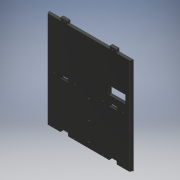
# Autodesk Inventor part: BA04
Saved by Autodesk Inventor 2017 (Build 210142000, 142)
## iProperties
Created: 2019-05-22
Part Number: BA04
Material: Wood (Cherry)
Document SubType Name: Modeling
Designer: Dell
Density: 0.63 g/cm^3
Appearance: Smooth - Black
Mass: 791.209 g
Surface Area: 2249.26 cm^2
Volume: 1255.89 cm^3
Author: Dell
Autodesk Inventor part; units mm, degrees
ref_plane "YZ Plane" through (0, 0, 0) normal (1, 0, 0) x (0, 1, 0)
ref_plane "XZ Plane" through (0, 0, 0) normal (0, 1, 0) x (-1, 0, 0)
ref_plane "XY Plane" through (0, 0, 0) normal (0, 0, 1) x (1, 0, 0)
sketch "Sketch1" plane through (0, 0, 0) normal (0, 0, 1) x (1, 0, 0)
  line L0 (0, 0) -> (303.5592, 0)
  line L1 (303.5592, 0) -> (455.3388, -262.89) construction
  line L2 (455.3388, -262.89) -> (404.5388, -350.8782)
  line L3 (404.5388, -350.8782) -> (-50.8, -87.9882) construction
  line L4 (-50.8, -87.9882) -> (0, 0) construction
  line L5 (0, 0) -> (5.4993, -9.525)
  line L6 (5.4993, -9.525) -> (298.06, -9.525)
  line L7 (298.06, -9.525) -> (303.5592, 0)
  dimension "d0" = 525.78
  dimension "d1" = 101.6
  dimension "d2" = 120
  dimension "d3" = 9.525
  dimension "d4" = 60
  dimension "d5" = 60
  constraints: 16 end point, 2 equal length, 2 horizontal, 2 perpendicular
  measures "d0" distance of L2.end L3.end
  measures "d1" distance of L3.end L0.start
  measures "d2" angle of L0 L4
  measures "d3" distance between parallel lines of L0 L6
  measures "d4" angle of L0 L5
  measures "d5" angle of L0 L7
extrude "Extrusion1" add sketch "Sketch1" along normal blind 346.075
sketch "Sketch2" plane through (5.4993, -9.525, 0) normal (0, -1, 0) x (1, 0, 0)
  line L0 (298.06, 346.075) -> (-5.4993, 346.075) projected
  line L1 (45.3007, 346.075) -> (70.7007, 346.075)
  line L2 (70.7007, 346.075) -> (70.7007, 355.6)
  line L3 (70.7007, 355.6) -> (45.3007, 355.6)
  line L4 (45.3007, 355.6) -> (45.3007, 346.075)
  line L5 (221.86, 346.075) -> (247.26, 346.075)
  line L6 (247.26, 346.075) -> (247.26, 355.6)
  line L7 (247.26, 355.6) -> (221.86, 355.6)
  line L8 (221.86, 355.6) -> (221.86, 346.075)
  line L9 (-5.4993, 0) -> (-5.4993, 346.075) projected
  line L10 (298.06, 0) -> (298.06, 346.075) projected
  circle A0 centre (58.0007, 350.8375) radius 2.25
  circle A1 centre (234.56, 350.8375) radius 2.25
  point P0 (58.0007, 355.6)
  point P1 (234.56, 355.6)
  point P2 (70.7007, 350.8375)
  point P3 (247.26, 350.8375)
  dimension "d8" = 25.4
  dimension "d9" = 9.525
  dimension "d10" = 25.4
  dimension "d11" = 9.525
  dimension "d12" = 50.8
  dimension "d13" = 50.8
  dimension "d16" = 4.5
  dimension "d17" = 4.5
  constraints: 16 end point, 4 midpoint, 4 parallel, 2 centre point, 2 horizontal, 2 horizontal alignment, 2 perpendicular, 2 point on line, 2 vertical alignment
  measures "d8" distance of L3.end L2.end
  measures "d9" distance of L2.end L1.end
  measures "d10" distance of L7.end L6.end
  measures "d11" distance of L6.end L5.end
  measures "d12" distance between parallel lines of L9 L4
  measures "d13" distance between parallel lines of L10 L6
  measures "d16" diameter of A0
  measures "d17" diameter of A1
extrude "Extrusion2" add sketch "Sketch2" against normal blind 9.525
ref_plane "Work Plane1" through (0, 0, 295.275) normal (0, 0, 1) x (1, 0, 0)
sketch "Sketch3" plane through (0, 0, 295.275) normal (0, 0, 1) x (1, 0, 0)
  line L0 (0, 0) -> (303.5592, 0) projected
  line L1 (0, 0) -> (0, -9.525)
  line L2 (298.06, -9.525) -> (5.4993, -9.525) projected
  line L3 (0, -9.525) -> (5.4993, -9.525)
  line L4 (5.4993, -9.525) -> (0, 0) projected
  constraints: 4 end point, 1 perpendicular, 1 vertical
extrude "Extrusion3" [suppressed]
ref_plane "Work Plane2" through (0, 0, 50.8) normal (0, 0, -1) x (-1, 0, 0)
sketch "Sketch4" plane through (0, 0, 50.8) normal (0, 0, -1) x (-1, 0, 0)
  line L0 (0, -12.7) -> (0, 0) projected
  line L1 (-7.3323, -12.7) -> (0, 0) projected
  line L2 (-7.3323, -12.7) -> (0, -12.7) projected
extrude "Extrusion4" [suppressed]
ref_plane "Work Plane3" through (0, 0, 173.0375) normal (0, 0, -1) x (-1, 0, 0)
sketch "Sketch5" plane through (0, 0, 173.0375) normal (0, 0, -1) x (-1, 0, 0)
  line L0 (0, 0) -> (0, -12.7) projected
  line L1 (0, -12.7) -> (-7.3323, -12.7) projected
  line L2 (0, 0) -> (-7.3323, -12.7) projected
extrude "Extrusion5" [suppressed]
ref_plane "Work Plane4" through (151.7796, -9.525, 346.075) normal (-1, 0, 0) x (0, 0, 1)
mirror "Mirror1" [suppressed]
sketch "Sketch6" plane through (0, 0, 0) normal (0, 0, -1) x (-1, 0, 0)
  line L0 (-76.9796, -9.525) -> (-76.9796, 0)
  line L1 (-76.9796, -4.7625) -> (-64.2796, -4.7625) construction
  circle A0 centre (-64.2796, -4.7625) radius 2.25
  line L2 (-64.2796, -4.7625) -> (-64.2796, 0) construction
  line L3 (-51.5796, -9.525) -> (-76.9796, -9.525)
  line L4 (-76.9796, 0) -> (-51.5796, 0)
  line L5 (-51.5796, 0) -> (-51.5796, -9.525)
  line L6 (-226.5796, 0) -> (-226.5796, -9.525)
  line L7 (-239.2796, 0) -> (-64.2796, 0) construction
  line L8 (-251.9796, 0) -> (-226.5796, 0)
  line L9 (-251.9796, -9.525) -> (-251.9796, 0)
  circle A1 centre (-239.2796, -4.7625) radius 2.25
  line L10 (-239.2796, -4.7625) -> (-239.2796, 0) construction
  line L11 (-239.2796, -4.7625) -> (-226.5796, -4.7625) construction
  line L12 (-226.5796, -9.525) -> (-251.9796, -9.525)
  line L13 (0, 0) -> (-303.5592, 0)
  line L14 (0, 0) -> (-303.5592, 0) projected
  line L15 (-298.06, -9.525) -> (-5.4993, -9.525) projected
  point P0 (-151.7796, 0)
  dimension "d26" = 25.4
  dimension "d29" = 25.4
  dimension "d30" = 175
  dimension "d31" = 4.5
  dimension "d32" = 4.5
  constraints: 28 end point, 7 midpoint, 6 perpendicular, 6 point on line, 4 parallel, 2 centre point
  measures "d26" distance of L0.end L5.start
  measures "d29" distance of L8.start L6.start
  measures "d30" distance of L7.start L2.end
  measures "d31" diameter of A1
  measures "d32" diameter of A0
extrude "Extrusion6" cut sketch "Sketch6" against normal blind 9.525 contours L0 L4 L5 L3 | L12 L9 L8 L6 | A0 | A1
sketch "Sketch7" plane through (227.3592, -9.525, 355.6) normal (0, -1, 0) x (1, 0, 0)
  line L0 (-175.7796, -178.275) -> (-150.3796, -178.275)
  line L1 (-150.3796, -178.275) -> (-150.3796, -187.8)
  line L2 (-150.3796, -187.8) -> (-175.7796, -187.8)
  line L3 (-175.7796, -187.8) -> (-175.7796, -178.275)
  line L4 (-0.7796, -178.275) -> (24.6204, -178.275)
  line L5 (24.6204, -178.275) -> (24.6204, -187.8)
  line L6 (24.6204, -187.8) -> (-0.7796, -187.8)
  line L7 (-0.7796, -187.8) -> (-0.7796, -178.275)
  line L8 (-175.7796, -346.075) -> (-150.3796, -346.075) projected
  line L9 (-0.7796, -346.075) -> (24.6204, -346.075) projected
  line L10 (-221.86, -9.525) -> (-176.5592, -9.525) projected
  point P0 (-227.3592, -355.6)
  point P1 (-163.0796, -187.8)
  point P2 (-163.0796, -346.075)
  point P3 (11.9204, -187.8)
  point P4 (11.9204, -346.075)
  dimension "d36" = 25.4
  dimension "d37" = 9.525
  dimension "d38" = 25.4
  dimension "d39" = 9.525
  dimension "d100" = 168.75
  constraints: 16 end point, 4 midpoint, 4 parallel, 2 horizontal, 2 perpendicular, 2 vertical alignment, 1 horizontal alignment
  measures "d36" distance of L1.end L2.end
  measures "d37" distance of L0.end L1.end
  measures "d38" distance of L5.end L6.end
  measures "d39" distance of L4.end L5.end
  measures "d100" distance between parallel lines of L10 L0
extrude "Extrusion7" cut sketch "Sketch7" against normal through all
sketch "Sketch8" plane through (227.3592, -9.525, 355.6) normal (0, -1, 0) x (1, 0, 0)
  line L0 (-150.3796, -355.6) -> (-0.7796, -355.6) construction
  line L1 (-100.9796, -355.6) -> (-50.1796, -355.6) construction
  line L2 (-50.1796, -355.6) -> (-50.1796, -178.275) construction
  line L3 (-50.1796, -178.275) -> (-100.9796, -178.275) construction
  line L4 (-100.9796, -178.275) -> (-100.9796, -355.6) construction
  circle A0 centre (-75.5796, -267.89) radius 4
  circle A1 centre (-75.5796, -200.18) radius 4
  circle A2 centre (-75.5796, -335.6) radius 4
  line L5 (-0.7796, -355.6) -> (-150.3796, -355.6)
  line L6 (-0.7796, -355.6) -> (-150.3796, -355.6) projected
  circle A3 centre (-126.3796, -183.0375) radius 2.25
  circle A4 centre (-126.3796, -350.8375) radius 2.25
  circle A5 centre (-24.7796, -350.8375) radius 2.25
  circle A6 centre (-24.7796, -183.0375) radius 2.25
  line L7 (-150.3796, -178.275) -> (-150.3796, -187.8) projected
  line L8 (-150.3796, -346.075) -> (-150.3796, -355.6) projected
  point P0 (-75.5796, -355.6)
  point P1 (-75.5796, -355.6)
  point P2 (-75.5796, -355.6)
  point P3 (-100.9796, -266.9375)
  point P4 (-150.3796, -183.0375)
  point P5 (-150.3796, -350.8375)
  dimension "d44" = 8
  dimension "d45" = 8
  dimension "d46" = 8
  dimension "d48" = 20
  dimension "d49" = 50.8
  dimension "d59" = 4.5
  dimension "d60" = 4.5
  dimension "d61" = 4.5
  dimension "d62" = 4.5
  dimension "d63" = 25.4
  dimension "d64" = 25.4
  dimension "d98" = 67.71
  dimension "d99" = 67.71
  constraints: 12 end point, 7 centre point, 7 midpoint, 5 horizontal alignment, 5 vertical alignment, 2 coincident, 2 parallel, 1 horizontal, 1 perpendicular, 1 point on line
  measures "d44" diameter of A0
  measures "d45" diameter of A1
  measures "d46" diameter of A2
  measures "d48" distance from line of L0 A2.centre
  measures "d49" distance of L2.end L3.end
  measures "d59" diameter of A3
  measures "d60" diameter of A4
  measures "d61" diameter of A5
  measures "d62" diameter of A6
  measures "d63" distance from line of A3.centre L4
  measures "d64" distance from line of A6.centre L2
  measures "d98" distance of A2.centre A0.centre
  measures "d99" distance of A0.centre A1.centre
extrude "Extrusion8" cut sketch "Sketch8" against normal through all
sketch "Sketch9" plane through (227.3592, -9.525, 355.6) normal (0, -1, 0) x (1, 0, 0)
  circle A0 centre (-198.8198, -183.0375) radius 2.25
  circle A1 centre (47.6606, -183.0375) radius 2.25
  circle A2 centre (-198.8198, -350.8375) radius 2.25
  circle A3 centre (47.6606, -350.8375) radius 2.25
  line L0 (-175.7796, -187.8) -> (-175.7796, -178.275) projected
  line L1 (-175.7796, -355.6) -> (-175.7796, -346.075) projected
  line L2 (24.6204, -346.075) -> (24.6204, -355.6) projected
  line L3 (-175.7796, -355.6) -> (-221.86, -355.6) projected
  line L4 (70.7007, -355.6) -> (24.6204, -355.6) projected
  line L5 (24.6204, -178.275) -> (24.6204, -187.8) projected
  point P0 (-227.3592, -355.6)
  point P1 (-175.7796, -183.0375)
  point P2 (-175.7796, -350.8375)
  point P3 (24.6204, -350.8375)
  point P4 (-198.8198, -355.6)
  point P5 (47.6606, -355.6)
  point P6 (24.6204, -183.0375)
  dimension "d52" = 4.5
  dimension "d54" = 4.5
  dimension "d55" = 4.5
  dimension "d56" = 4.5
  constraints: 6 midpoint, 4 centre point, 4 horizontal alignment, 4 vertical alignment
  measures "d52" diameter of A0
  measures "d54" diameter of A1
  measures "d55" diameter of A2
  measures "d56" diameter of A3
extrude "Extrusion9" cut sketch "Sketch9" against normal through all
sketch "Sketch12" plane through (76.2, 0, 346.075) normal (0, 1, 0) x (1, 0, 0)
  line L0 (208.0635, 143.75) -> (178.0635, 143.75)
  line L1 (178.0635, 143.75) -> (178.0635, 128.75)
  line L2 (178.0635, 128.75) -> (208.0635, 128.75)
  line L3 (208.0635, 128.75) -> (208.0635, 143.75)
  line L4 (0.7796, 168.75) -> (-24.6204, 168.75) projected
  line L5 (221.86, 346.075) -> (221.86, 0) projected
  point P0 (-76.2, 346.075)
  dimension "d70" = 30
  dimension "d71" = 15
  dimension "d72" = 25
  dimension "d76" = 13.7965
  constraints: 8 end point, 2 parallel, 1 horizontal, 1 perpendicular
  measures "d70" distance of L2.end L1.end
  measures "d71" distance of L1.end L0.end
  measures "d72" distance between parallel lines of L4 L0
  measures "d76" distance between parallel lines of L5 L3
extrude "Extrusion11" cut sketch "Sketch12" against normal through all
sketch "Sketch13" plane through (227.3592, -9.525, 355.6) normal (0, -1, 0) x (1, 0, 0)
  line L0 (26.9043, -153.275) -> (56.9043, -153.275) projected
  line L1 (56.9043, -153.275) -> (-3.0957, -153.275)
  line L2 (-3.0957, -153.275) -> (-3.0957, -123.275)
  line L3 (-3.0957, -123.275) -> (56.9043, -123.275)
  line L4 (56.9043, -123.275) -> (56.9043, -153.275)
  point P0 (-227.3592, -355.6)
  dimension "d77" = 30
  dimension "d78" = 60
  constraints: 8 end point, 2 parallel, 1 horizontal, 1 perpendicular
  measures "d77" distance of L3.end L0.end
  measures "d78" distance of L0.end L1.end
extrude "Extrusion12" cut sketch "Sketch13" against normal through all
sketch "Sketch16" plane through (227.3592, -9.525, 355.6) normal (0, -1, 0) x (1, 0, 0)
  line L0 (-175.7796, -355.6) -> (-221.86, -355.6) projected
  line L1 (-177.0496, -355.6) -> (-149.1096, -355.6)
  line L2 (-149.1096, -355.6) -> (-149.1096, -344.805)
  line L3 (-149.1096, -344.805) -> (-177.0496, -344.805)
  line L4 (-177.0496, -344.805) -> (-177.0496, -355.6)
  line L5 (-150.3796, -355.6) -> (-0.7796, -355.6) projected
  line L6 (-2.0496, -355.6) -> (25.8904, -355.6)
  line L7 (25.8904, -355.6) -> (25.8904, -344.805)
  line L8 (25.8904, -344.805) -> (-2.0496, -344.805)
  line L9 (-2.0496, -344.805) -> (-2.0496, -355.6)
  line L10 (-177.0496, -177.005) -> (-149.1096, -177.005)
  line L11 (-149.1096, -177.005) -> (-149.1096, -189.07)
  line L12 (-149.1096, -189.07) -> (-177.0496, -189.07)
  line L13 (-177.0496, -189.07) -> (-177.0496, -177.005)
  line L14 (-2.0496, -177.005) -> (25.8904, -177.005)
  line L15 (25.8904, -177.005) -> (25.8904, -189.07)
  line L16 (25.8904, -189.07) -> (-2.0496, -189.07)
  line L17 (-2.0496, -189.07) -> (-2.0496, -177.005)
  line L18 (-150.3796, -178.275) -> (-150.3796, -187.8) projected
  line L19 (-0.7796, -187.8) -> (-0.7796, -178.275) projected
  line L20 (-175.7796, -346.075) -> (-150.3796, -346.075) projected
  line L21 (-0.7796, -346.075) -> (24.6204, -346.075) projected
  line L22 (24.6204, -187.8) -> (-0.7796, -187.8) projected
  line L23 (-150.3796, -187.8) -> (-175.7796, -187.8) projected
  line L24 (-150.3796, -346.075) -> (-150.3796, -355.6) projected
  circle A0 centre (-178.8043, -7.2799) radius 3.175
  circle A1 centre (-148.9142, -7.2799) radius 3.175
  circle A2 centre (-2.2451, -7.2799) radius 3.175
  circle A3 centre (27.6451, -7.2799) radius 3.175
  line L25 (-176.5592, -9.525) -> (-178.8043, -7.2799)
  line L26 (-176.5592, 0) -> (-176.5592, -9.525) projected
  point P0 (-227.3592, -355.6)
  point P1 (-150.3796, -183.0375)
  point P2 (-149.1096, -183.0375)
  point P3 (-2.0496, -183.0375)
  point P4 (-0.7796, -183.0375)
  point P5 (-163.0796, -346.075)
  point P6 (-163.0796, -344.805)
  point P7 (11.9204, -346.075)
  point P8 (11.9204, -344.805)
  point P9 (11.9204, -187.8)
  point P10 (11.9204, -189.07)
  point P11 (-163.0796, -187.8)
  point P12 (-163.0796, -189.07)
  point P13 (-151.1592, -9.525)
  point P14 (0, -9.525)
  point P15 (25.4, -9.525)
  dimension "d93" = 6.35
  dimension "d94" = 6.35
  dimension "d95" = 6.35
  dimension "d96" = 6.35
  dimension "d83" = 1.27
  dimension "d84" = 1.27
  dimension "d85" = 1.27
  dimension "d86" = 1.27
  dimension "d87" = 1.27
  dimension "d97" = 45
  constraints: 34 end point, 12 midpoint, 8 horizontal alignment, 8 parallel, 4 horizontal, 4 perpendicular, 4 point on line, 4 vertical alignment, 1 coincident, 12 other
  measures "d83" distance between parallel lines of L11 L18
  measures "d84" distance between parallel lines of L23 L12
  measures "d85" distance between parallel lines of L19 L17
  measures "d86" distance between parallel lines of L2 L24
  measures "d87" distance between parallel lines of L3 L20
  measures "d97" angle of L25 L26
extrude "Extrusion14" cut sketch "Sketch16" against normal through all
sketch "Sketch17" plane through (227.3592, -9.525, 355.6) normal (0, -1, 0) x (1, 0, 0)
  line L0 (-176.5592, -9.525) -> (-176.5592, 0) projected
  line L1 (-176.5592, 0) -> (-151.1592, 0)
  line L2 (-151.1592, 0) -> (-151.1592, 1.27)
  line L3 (-151.1592, 1.27) -> (-176.5592, 1.27)
  line L4 (-176.5592, 1.27) -> (-176.5592, 0)
  line L5 (25.4, 0) -> (25.4, -9.525) projected
  line L6 (25.4, 0) -> (0, 0)
  line L7 (0, 0) -> (0, 1.27)
  line L8 (0, 1.27) -> (25.4, 1.27)
  line L9 (25.4, 1.27) -> (25.4, 0)
  point P0 (-227.3592, -355.6)
  point P1 (-151.1592, 0)
  dimension "d90" = 1.27
  constraints: 16 end point, 4 parallel, 2 coincident, 2 horizontal, 2 perpendicular, 1 point on line
  measures "d90" distance of L3.end L0.end
extrude "Extrusion15" add sketch "Sketch17" against normal up to surface (9.525 mm away) from surface at 0
sketch "Sketch18" plane through (298.06, -9.525, 0) normal (0, -1, 0) x (1, 0, 0)
  line L0 (-247.26, 350.5651) -> (-247.26, 356.87) projected
  arc A0 (-251.7501, 346.075) -> (-247.26, 350.5651) centre (-249.505, 348.3201) ccw projected
  line L1 (-247.26, 356.87) -> (-247.895, 356.87)
  line L2 (-247.895, 356.87) -> (-247.895, 345.5836)
  line L3 (-247.895, 345.5836) -> (-247.26, 345.5836)
  line L4 (-247.26, 345.5836) -> (-247.26, 356.87)
  arc A1 (-221.86, 350.5651) -> (-217.3698, 346.075) centre (-219.6149, 348.3201) ccw projected
  line L5 (-221.86, 356.87) -> (-222.495, 356.87)
  line L6 (-222.495, 356.87) -> (-222.495, 346.9837)
  line L7 (-222.495, 346.9837) -> (-221.86, 346.9837)
  line L8 (-221.86, 346.9837) -> (-221.86, 356.87)
  line L9 (-70.7007, 350.5651) -> (-70.7007, 356.87) projected
  arc A2 (-75.1909, 346.075) -> (-70.7007, 350.5651) centre (-72.9458, 348.3201) ccw projected
  line L10 (-70.7007, 356.87) -> (-70.0657, 356.87)
  line L11 (-70.0657, 356.87) -> (-70.0657, 349.6564)
  line L12 (-70.0657, 349.6564) -> (-70.7007, 349.6564)
  line L13 (-70.7007, 349.6564) -> (-70.7007, 356.87)
  line L14 (-45.3007, 350.5651) -> (-45.3007, 356.87) projected
  arc A3 (-45.3007, 350.5651) -> (-40.8106, 346.075) centre (-43.0557, 348.3201) ccw projected
  line L15 (-45.3007, 356.87) -> (-45.9357, 356.87)
  line L16 (-45.9357, 356.87) -> (-45.9357, 349.6564)
  line L17 (-45.9357, 349.6564) -> (-45.3007, 349.6564)
  line L18 (-45.3007, 349.6564) -> (-45.3007, 356.87)
  point P0 (-298.06, 0)
  dimension "d101" = 0.635
  dimension "d102" = 0.635
  dimension "d103" = 0.635
  dimension "d104" = 0.635
  constraints: 32 end point, 8 parallel, 4 horizontal, 4 perpendicular, 4 point on circle, 1 coincident, 1 point on line
  measures "d101" distance between parallel lines of L14 L16
  measures "d102" distance between parallel lines of L13 L11
  measures "d103" distance between parallel lines of L8 L6
  measures "d104" distance between parallel lines of L0 L2
extrude "Extrusion16" cut sketch "Sketch18" against normal through all contours L4 A0 L2 L1 L0 | L4 L3 A0 | L8 L7 L6 A1 | A1 L6 L5 L8 | L9 L10 L11 A2 | A2 L12 L13 | A3 L16 L15 L14 | L18 L17 A3
equation "\"d3\" = Panel_Thickness"
equation "\"d9\" = Panel_Thickness"
equation "\"d11\" = Panel_Thickness"
equation "\"d14\" = Panel_Thickness"
equation "\"d34\" = Panel_Thickness"
equation "\"d37\" = Panel_Thickness"
equation "\"d39\" = d37"
equation "\"d93\" = Tool_Dia"
equation "\"d94\" = Tool_Dia"
equation "\"d95\" = d94"
equation "\"d96\" = d94"
equation "\"d83\" = Fit_Tolerance"
equation "\"d84\" = Fit_Tolerance"
equation "\"d85\" = Fit_Tolerance"
equation "\"d86\" = Fit_Tolerance"
equation "\"d87\" = Fit_Tolerance"
equation "\"d90\" = Fit_Tolerance"
equation "\"d101\" = 0.5 * Fit_Tolerance"
equation "\"d102\" = 0.5 * Fit_Tolerance"
equation "\"d103\" = 0.5 * Fit_Tolerance"
equation "\"d104\" = 0.5 * Fit_Tolerance"
equation "\"Panel_Thickness\" = 9.525"
equation "\"Fit_Tolerance\" = 1.27"
equation "\"Tool_Dia\" = 6.35"
body "Solid1"
